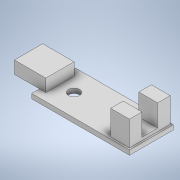
# Autodesk Inventor part: irencoder_footprint
Saved by Autodesk Inventor 2021 (Build 250183000, 183)
## iProperties
Created: 2021-12-11
Part Number: irencoder_footprint
Material: Generic
Document SubType Name: Modeling
Designer: Juan M. Casillas
Density: 1 g/cm^3
Appearance: Default
Author: Juan M. Casillas
Autodesk Inventor part; units mm, degrees
ref_plane "YZ Plane" through (0, 0, 0) normal (1, 0, 0) x (0, 1, 0)
ref_plane "XZ Plane" through (0, 0, 0) normal (0, 1, 0) x (-1, 0, 0)
ref_plane "XY Plane" through (0, 0, 0) normal (0, 0, 1) x (1, 0, 0)
sketch "Sketch1" plane through (0, 0, 0) normal (0, 1, 0) x (-1, 0, 0)
  line L0 (15.6, 7) -> (-15.6, 7)
  line L1 (-15.6, 7) -> (-15.6, -7)
  line L2 (-15.6, -7) -> (15.6, -7)
  line L3 (15.6, -7) -> (15.6, 7)
  line L4 (15.6, 7) -> (-15.6, -7) construction
  line L5 (-15.6, 7) -> (15.6, -7) construction
  point P0 (0, 0)
  dimension "d0" = 31.2
  dimension "d1" = 14
  constraints: 12 end point, 2 midpoint, 2 parallel, 1 horizontal, 1 perpendicular
  measures "d0" distance of L2.end L1.end
  measures "d1" distance of L1.end L0.end
extrude "Extrusion1" add sketch "Sketch1" along normal blind 1.5
sketch "Sketch2" plane through (0, 1.5, 0) normal (0, 1, 0) x (1, 0, 0)
  line L0 (9.1, -6.5) -> (15.1, -6.5)
  line L1 (15.1, -6.5) -> (15.1, 6.5)
  line L2 (15.1, 6.5) -> (9.1, 6.5)
  line L3 (9.1, 6.5) -> (9.1, -6.5)
  line L4 (9.1, -6.5) -> (15.1, 6.5) construction
  line L5 (15.1, -6.5) -> (9.1, 6.5) construction
  line L6 (15.6, 7) -> (-15.6, 7) projected
  line L7 (15.6, -7) -> (15.6, 7) projected
  point P0 (0, 0)
  point P1 (12.1, 0)
  point P2 (15.1, 0)
  point P3 (15.1, 0)
  dimension "d4" = 6
  dimension "d5" = 13
  dimension "d6" = 7
  dimension "d7" = 0.5
  constraints: 12 end point, 3 midpoint, 2 parallel, 1 coincident, 1 horizontal, 1 perpendicular
  measures "d4" distance of L2.end L1.end
  measures "d5" distance of L1.end L0.end
  measures "d6" distance from line of L6 point (15.1, 0)
  measures "d7" distance from line of L7 point (15.1, 0)
extrude "Extrusion2" add sketch "Sketch2" along normal blind 8
sketch "Sketch3" plane through (0, 9.5, 0) normal (0, 1, 0) x (1, 0, 0)
  line L0 (15.1, -6.5) -> (15.1, 6.5) construction
  line L1 (15.1, 6.5) -> (9.1, 6.5) construction
  line L2 (9.1, 6.5) -> (9.1, -6.5) construction
  line L3 (9.1, -6.5) -> (15.1, -6.5) construction
  line L4 (9.1, -6.5) -> (15.1, -6.5)
  line L5 (15.1, -6.5) -> (15.1, -2.5)
  line L6 (15.1, -2.5) -> (9.1, -2.5)
  line L7 (9.1, -2.5) -> (9.1, -6.5)
  line L8 (9.1, 6.5) -> (15.1, 6.5)
  line L9 (15.1, 6.5) -> (15.1, 2.5)
  line L10 (15.1, 2.5) -> (9.1, 2.5)
  line L11 (9.1, 2.5) -> (9.1, 6.5)
  line L12 (9.1, -2.5) -> (15.1, -2.5)
  line L13 (15.1, -2.5) -> (15.1, 2.5)
  line L14 (15.1, 2.5) -> (9.1, 2.5)
  line L15 (9.1, 2.5) -> (9.1, -2.5)
  point P0 (0, 0)
  dimension "d10" = 4
  dimension "d11" = 4
  constraints: 24 end point, 6 parallel, 3 horizontal, 3 perpendicular, 2 point on line
  measures "d10" distance of L5.end L4.end
  measures "d11" distance of L8.end L9.end
extrude "Extrusion3" cut sketch "Sketch3" against normal blind 7 contours L15 L10 L13 L6
sketch "Sketch4" plane through (0, 1.5, 0) normal (0, 1, 0) x (1, 0, 0)
  line L0 (-15.6, 7) -> (-15.6, -7) construction
  line L1 (-15.6, 0) -> (-9.1, 0) construction
  point P0 (0, 0)
  dimension "d14" = 6.5
  constraints: 2 end point, 1 coincident, 1 horizontal, 1 midpoint
  measures "d14" distance of L1.start L1.end
hole "Hole1" at (-9.1, 1.5, 0) direction (0, -1, 0) diameter 3.5 end through all
sketch "Sketch5" plane through (0, 1.5, 0) normal (0, 1, 0) x (1, 0, 0)
  circle A0 centre (-9.1, 0) radius 1.75 construction
  line L0 (15.1, -6.5) -> (9.1, -6.5) construction
  line L1 (9.1, -6.5) -> (9.1, 6.5) construction
  line L2 (9.1, 6.5) -> (15.1, 6.5) construction
  line L3 (15.1, 6.5) -> (15.1, -6.5) construction
  line L4 (15.6, -7) -> (15.6, 7) construction
  line L5 (15.6, 7) -> (-15.6, 7) construction
  line L6 (-15.6, 7) -> (-15.6, -7) construction
  line L7 (-15.6, -7) -> (15.6, -7) construction
  line L8 (-23.6, 4.5) -> (-13.6, 4.5)
  line L9 (-13.6, 4.5) -> (-13.6, -4.5)
  line L10 (-13.6, -4.5) -> (-23.6, -4.5)
  line L11 (-23.6, -4.5) -> (-23.6, 4.5)
  line L12 (-13.6, 7) -> (-13.6, -7) construction
  point P0 (0, 0)
  point P1 (-13.6, 0)
  dimension "d22" = 10
  dimension "d23" = 9
  dimension "d24" = 2
  constraints: 10 end point, 2 midpoint, 2 parallel, 2 perpendicular, 2 point on line, 1 horizontal
  measures "d22" distance of L9.end L10.end
  measures "d23" distance of L8.end L9.end
  measures "d24" distance between parallel lines of L6 L12
extrude "Extrusion4" add sketch "Sketch5" along normal blind 4
body "Solid1"
